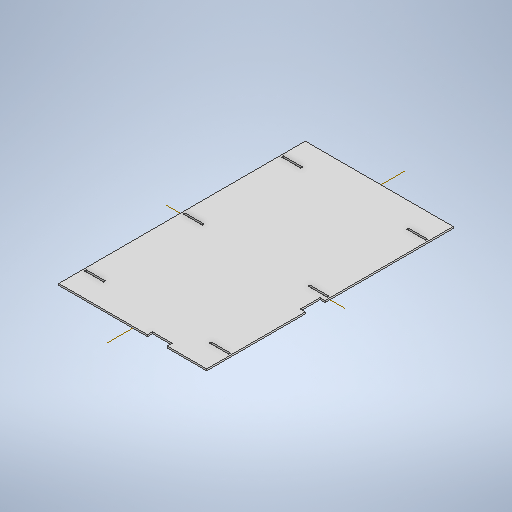
# Autodesk Inventor part: 부품1
Saved by Autodesk Inventor 2025 (Build 290162000, 162)
## iProperties
Created: 2024-04-04
Part Number: 부품1
Material: 일반
Document SubType Name: Modeling
Designer: gmsee
Density: 1 g/cm^3
Appearance: 기본값
Author: gmsee
Autodesk Inventor part; units mm, degrees
ref_plane "YZ Plane" through (0, 0, 0) normal (1, 0, 0) x (0, 1, 0)
ref_plane "XZ Plane" through (0, 0, 0) normal (0, 1, 0) x (-1, 0, 0)
ref_plane "XY Plane" through (0, 0, 0) normal (0, 0, 1) x (1, 0, 0)
sketch "스케치1" plane through (0, 0, 0) normal (0, 1, 0) x (-1, 0, 0)
  line L0 (150, 0) -> (150, -250)
  line L1 (150, -250) -> (0, -250)
  line L2 (216.1767, 0) -> (-247.0601, 0) projected
  line L3 (0, -350) -> (0, 350) projected
  line L4 (100, 0) -> (100, -250) construction
  line L5 (107.4, -198.15) -> (107.4, -201.85)
  line L6 (107.4, -201.85) -> (146.1, -201.85)
  line L7 (146.1, -198.15) -> (107.4, -198.15)
  line L8 (146.1, -201.85) -> (146.1, -198.15)
  line L9 (146.1, 0) -> (146.1, -1.85)
  line L10 (146.1, -1.85) -> (107.4, -1.85)
  line L11 (107.4, -1.85) -> (107.4, 0)
  line L12 (150, 0) -> (150, 250)
  line L13 (150, 250) -> (0, 250)
  line L14 (100, 0) -> (100, 250) construction
  line L15 (146.1, 198.15) -> (107.4, 198.15)
  line L16 (146.1, 201.85) -> (146.1, 198.15)
  line L17 (107.4, 201.85) -> (146.1, 201.85)
  line L18 (107.4, 198.15) -> (107.4, 201.85)
  line L19 (146.1, 0) -> (146.1, 1.85)
  line L20 (146.1, 1.85) -> (107.4, 1.85)
  line L21 (107.4, 1.85) -> (107.4, 0)
  line L22 (-150, -250) -> (0, -250)
  line L23 (-100, 0) -> (-100, -250) construction
  line L24 (-146.1, -198.15) -> (-107.4, -198.15)
  line L25 (-146.1, -201.85) -> (-146.1, -198.15)
  line L26 (-107.4, -201.85) -> (-146.1, -201.85)
  line L27 (-107.4, -198.15) -> (-107.4, -201.85)
  line L28 (-146.1, 0) -> (-146.1, -1.85)
  line L29 (-146.1, -1.85) -> (-107.4, -1.85)
  line L30 (-107.4, -1.85) -> (-107.4, 0)
  line L31 (-146.1, 1.85) -> (-107.4, 1.85)
  line L32 (-146.1, 0) -> (-146.1, 1.85)
  line L33 (-107.4, 1.85) -> (-107.4, 0)
  line L34 (-100, 0) -> (-100, 250) construction
  line L35 (-146.1, 198.15) -> (-107.4, 198.15)
  line L36 (-107.4, 198.15) -> (-107.4, 201.85)
  line L37 (-146.1, 201.85) -> (-146.1, 198.15)
  line L38 (-107.4, 201.85) -> (-146.1, 201.85)
  line L39 (-150, -250) -> (-150, 10)
  line L40 (-150, -250) -> (-180.8834, -250)
  line L41 (-150, 10) -> (-139.9, 10)
  line L42 (-139.9, 10) -> (-139.9, 50)
  line L43 (-139.9, 50) -> (-150, 50)
  line L44 (-150, 0) -> (-150, 10)
  line L45 (-150, 50) -> (-150, 250)
  line L46 (-30, 250) -> (-30, 239.9)
  line L47 (-30, 239.9) -> (-70, 239.9)
  line L48 (-70, 239.9) -> (-70, 250)
  line L49 (-150, 250) -> (-70, 250)
  line L50 (-30, 250) -> (0, 250)
  point P0 (0, 0)
  dimension "d2" = 250
  dimension "d3" = 150
  dimension "d4" = 50
  dimension "d13" = 38.7
  dimension "d14" = 3.7
  dimension "d15" = 48.15
  dimension "d16" = 1.85
  dimension "d17" = 38.7
  dimension "d18" = 7.4
  dimension "d19" = 7.4
  dimension "d50" = 10.1
  dimension "d51" = 10
  dimension "d52" = 40
  dimension "d54" = 30
  dimension "d55" = 40
  dimension "d57" = 10.1
  constraints: 98 end point, 29 symmetric about line, 12 perpendicular, 5 point on line, 3 parallel, 2 horizontal, 2 vertical
  measures "d2" distance of L0.start L0.end
  measures "d3" distance of L0.end L1.end
  measures "d4" distance between parallel lines of L0 L4
  measures "d13" distance of L6.start L8.start
  measures "d14" distance of L7.end L6.start
  measures "d15" distance between parallel lines of L1 L6
  measures "d16" distance of L9.start L9.end
  measures "d17" distance of L9.end L10.end
  measures "d18" distance between parallel lines of L4 L11
  measures "d19" distance between parallel lines of L4 L5
  measures "d50" distance of L39.end L41.end
  measures "d51" distance between parallel lines of L2 L41
  measures "d52" distance between parallel lines of L41 L43
  measures "d54" distance between parallel lines of L3 L46
  measures "d55" distance of L46.end L47.end
  measures "d57" distance of L47.end L48.end
extrude "돌출1" add sketch "스케치1" along normal blind 3.5 contours L0 L1 L3 L2 L11 L10 L9 | L2 L19 L20 L21 L3 L13 L12 | L22 L39 L2 L28 L29 L30 L3 | L3 L2 L33 L31 L32 L39 L41 L42 L43 L45 L49 L48 L47 L46 L50
